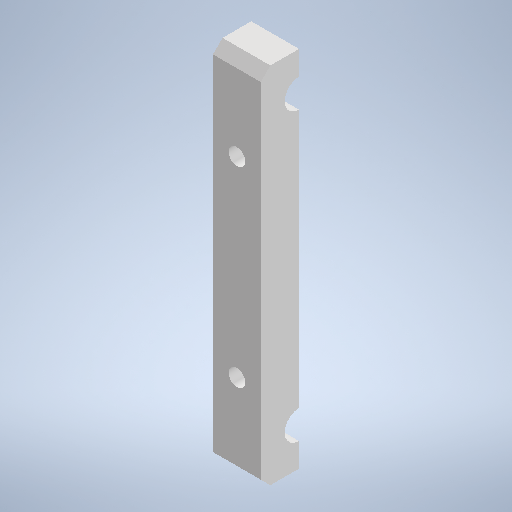
# Autodesk Inventor part: 6_2xclamp_main
Saved by Autodesk Inventor 2025.1 (Build 291241000, 241)
## iProperties
Created: 2024-10-31
Part Number: 6_2xclamp_main
Material: Ogólny
Document SubType Name: Modeling
Designer: PC
Density: 1 g/cm^3
Appearance: Domyślna
Author: PC
Autodesk Inventor part; units mm, degrees
ref_plane "YZ Plane" through (0, 0, 0) normal (1, 0, 0) x (0, 1, 0)
ref_plane "XZ Plane" through (0, 0, 0) normal (0, 1, 0) x (-1, 0, 0)
ref_plane "XY Plane" through (0, 0, 0) normal (0, 0, 1) x (1, 0, 0)
sketch "Szkic1" plane through (0, 0, 0) normal (1, 0, 0) x (0, 1, 0)
  circle A0 centre (0, 0) radius 3 construction
  circle A1 centre (60, 0) radius 3 construction
  arc A2 (63, 0) -> (57, 0) centre (60, 0) ccw
  arc A3 (3, 0) -> (-3, 0) centre (0, 0) ccw
  line L0 (68, 0) -> (68, 8)
  line L1 (68, 8) -> (-8, 8)
  line L2 (-8, 8) -> (-8, 0)
  line L3 (63, 0) -> (68, 0)
  line L4 (-8, 0) -> (-3, 0)
  line L5 (3, 0) -> (57, 0)
  point P0 (-5.5, 0)
  dimension "d0" = 6
  dimension "d1" = 6
  dimension "d2" = 60
  dimension "d3" = 6
  dimension "d4" = 5
  dimension "d5" = 8
  constraints: 12 end point, 4 centre point, 4 parallel, 4 point on circle, 3 coincident, 3 horizontal, 3 perpendicular, 1 collinear, 1 concentric, 1 midpoint
  measures "d0" diameter of A0
  measures "d1" diameter of A1
  measures "d2" distance of point (0, 0) A1.centre
  measures "d3" diameter of A3
  measures "d4" distance of L3.start L0.start
  measures "d5" distance from line of point (-5.5, 0) L1
extrude "Wyciągnięcie proste1" add sketch "Szkic1" along normal blind 10
sketch "Szkic2" plane through (0, 3, 0) normal (0, 0, -1) x (-1, 0, 0)
  line L0 (0, 65) -> (-10, 65) construction
  line L1 (-5, 65) -> (-5, -11.1641) construction
  line L2 (-10, 65) -> (-10, -11) construction
  line L3 (-10, 27) -> (0, 27) construction
  line L4 (0, 65) -> (0, -11) construction
  circle A0 centre (-5, 47) radius 1.75
  circle A1 centre (-5, 7) radius 1.75
  circle A2 centre (-5, 37) radius 1.75
  circle A3 centre (-5, 17) radius 1.75
  point P0 (0, -3)
  dimension "d8" = 3.5
  dimension "d9" = 20
  dimension "d15" = 3.5
  dimension "d16" = 10
  constraints: 4 centre point, 4 end point, 3 midpoint, 2 point on line, 2 symmetric about line, 1 vertical, 2 other
  measures "d8" diameter of A0
  measures "d9" distance from line of L3 A0.centre
  measures "d15" diameter of A2
  measures "d16" distance from line of L3 A2.centre
extrude "Wyciągnięcie proste2" cut sketch "Szkic2" against normal up to next contours A0 | A1
chamfer "Faza1" distance 2 angle 45 2 edges at (5, 68, 8) (5, -8, 8)
